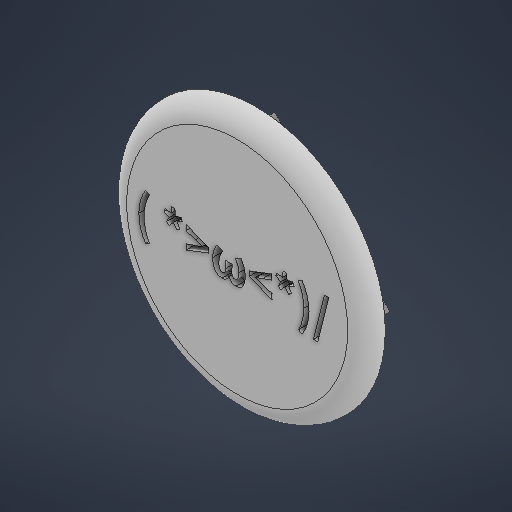
# Autodesk Inventor part: Part10
Saved by Autodesk Inventor 2026 (Build 300175000, 175)
## iProperties
Created: 2025-10-26
Part Number: Part10
Material: 一般
Document SubType Name: Modeling
Designer: masak
Density: 1 g/cm^3
Appearance: 既定
Author: masak
Autodesk Inventor part; units mm, degrees
ref_plane "YZ Plane" through (0, 0, 0) normal (1, 0, 0) x (0, 1, 0)
ref_plane "XZ Plane" through (0, 0, 0) normal (0, 1, 0) x (-1, 0, 0)
ref_plane "XY Plane" through (0, 0, 0) normal (0, 0, 1) x (1, 0, 0)
sketch "スケッチ1" plane through (0, 0, 0) normal (0, 0, 1) x (1, 0, 0)
  line L0 (23, 24.5) -> (3, 24.5) projected
  line L1 (23, 24.5) -> (3, 24.5) construction
  line L2 (23, 24.5) -> (3, 24.5)
  line L3 (23, 24.5) -> (3, 24.5)
  line L4 (23, 24.5) -> (3, 24.5)
  line L5 (23, 24.5) -> (3, 24.5) construction
  line L6 (13, 14.5) -> (3, 24.5) projected
  line L7 (3, 1.5) -> (13, 11.5) projected
  line L8 (11.5, 13) -> (1.5, 3) projected
  line L9 (1.5, 23) -> (11.5, 13) projected
  line L10 (1.5, 3) -> (1.5, 23) projected
  line L11 (0, 0) -> (0, 26) projected
  line L12 (0, 26) -> (50.5, 26) projected
  line L13 (50.5, 0) -> (0, 0) projected
  line L14 (0, 0) -> (-26, 0)
  line L15 (-26, 0) -> (-26, 26)
  line L16 (-26, 26) -> (0, 26)
  line L17 (0, 26) -> (0, 0)
  line L18 (-26, 0) -> (0, 26)
  line L19 (0, 0) -> (-26, 26)
  circle A0 centre (-13, 13) radius 27.5
  dimension "d0" = 26
  constraints: 18 end point, 2 parallel, 2 perpendicular, 1 centre point, 1 coincident, 1 horizontal, 1 midpoint
  measures "d0" distance of L15.end L16.end
extrude "押し出し1" add sketch "スケッチ1" along normal blind 4 contours L8 L10 L9 | L19 L18 L11 | L11 L12 A0 L13 | L13 A0 L12 L16 L15 L14 | L14 L18 L19 | L18 L19 L16 | L15 L19 L18
sketch "スケッチ2" plane through (-13, 13, 0) normal (0, 0, -1) x (-1, 0, 0)
  line L0 (-24.5, 0) -> (-14.5, 10) projected
  line L1 (-14.5, 10) -> (-14.5, -10) projected
  line L2 (-14.5, -10) -> (-24.5, 0) projected
  line L3 (-14.5, 10) -> (-14.5, -10)
  line L4 (-24.5, 0) -> (-14.5, 10)
  line L5 (-24.5, 0) -> (-14.5, -10)
  line L6 (-10, -14.5) -> (10, -14.5)
  line L7 (0, -24.5) -> (-10, -14.5)
  line L8 (0, -24.5) -> (10, -14.5)
  line L9 (14.5, -10) -> (14.5, 10)
  line L10 (24.5, 0) -> (14.5, -10)
  line L11 (24.5, 0) -> (14.5, 10)
  line L12 (10, 14.5) -> (-10, 14.5)
  line L13 (0, 24.5) -> (10, 14.5)
  line L14 (0, 24.5) -> (-10, 14.5)
  point P0 (-13, -13)
  point P1 (0, 0)
  dimension "d5" = 360
  constraints: 24 end point, 1 perpendicular, 1 vertical, 25 other
fillet "フィレット1" radius 4 1 edges at (-40.5, 13, 4)
extrude "押し出し2" add sketch "スケッチ2" along normal blind 4
sketch "スケッチ3" plane through (-13, 13, 4) normal (0, 0, 1) x (1, 0, 0)
  line L0 (-21.7114, 4.3311) -> (23.7979, 4.3311) construction
  line L1 (23.7979, 4.3311) -> (23.7979, -14.3854) construction
  line L2 (23.7979, -14.3854) -> (-21.7114, -14.3854) construction
  line L3 (-21.7114, -14.3854) -> (-21.7114, 4.3311) construction
  line L4 (-19.5093, -5.4449) -> (-18.6418, -5.0778)
  spline S0 degree 2 poles (-18.6418, -5.0778) (-19.229, -4.0369) (-19.7895, -1.728) (-19.7895, -0.5535) knots 0 0 0 1 2 2 2
  spline S1 degree 2 poles (-19.7895, -0.5535) (-19.7895, 0.6076) (-19.229, 2.9164) (-18.6418, 3.9574) knots 0 0 0 1 2 2 2
  line L5 (-18.6418, 3.9574) -> (-19.5093, 4.3244)
  spline S2 degree 2 poles (-19.5093, 4.3244) (-20.1766, 3.2434) (-20.9039, 0.8478) (-20.9106, -0.5535) knots 0 0 0 1 2 2 2
  spline S3 degree 2 poles (-20.9106, -0.5535) (-20.9039, -1.9682) (-20.1766, -4.3572) (-19.5093, -5.4449) knots 0 0 0 1 2 2 2
  line L6 (-14.4444, 0.4074) -> (-13.617, 1.3549)
  line L7 (-13.617, 1.3549) -> (-12.7895, 0.4074)
  line L8 (-12.7895, 0.4074) -> (-12.1823, 0.8411)
  line L9 (-12.1823, 0.8411) -> (-12.8229, 1.9155)
  line L10 (-12.8229, 1.9155) -> (-11.6952, 2.416)
  line L11 (-11.6952, 2.416) -> (-11.922, 3.1166)
  line L12 (-11.922, 3.1166) -> (-13.1299, 2.843)
  line L13 (-13.1299, 2.843) -> (-13.2433, 4.0909)
  line L14 (-13.2433, 4.0909) -> (-13.984, 4.0909)
  line L15 (-13.984, 4.0909) -> (-14.1041, 2.8564)
  line L16 (-14.1041, 2.8564) -> (-15.3119, 3.1166)
  line L17 (-15.3119, 3.1166) -> (-15.5388, 2.416)
  line L18 (-15.5388, 2.416) -> (-14.4177, 1.9155)
  line L19 (-14.4177, 1.9155) -> (-15.0383, 0.8411)
  line L20 (-15.0383, 0.8411) -> (-14.4444, 0.4074)
  line L21 (-10.8744, -2.3486) -> (-6.0364, -0.4801)
  line L22 (-6.0364, -0.4801) -> (-6.0364, 0.5141)
  line L23 (-6.0364, 0.5141) -> (-10.881, 2.3826)
  line L24 (-10.881, 2.3826) -> (-10.881, 1.2282)
  line L25 (-10.881, 1.2282) -> (-8.8858, 0.5475)
  line L26 (-8.8858, 0.5475) -> (-7.4444, 0.0404)
  line L27 (-7.4444, 0.0404) -> (-7.4444, 0.0003)
  line L28 (-7.4444, 0.0003) -> (-8.8858, -0.5135)
  line L29 (-8.8858, -0.5135) -> (-10.881, -1.1941)
  line L30 (-10.881, -1.1941) -> (-10.8744, -2.3486)
  spline S4 degree 2 poles (-3.2137, -3.6698) (-2.74, -3.6765) (-1.9926, -3.2094) (-1.779, -2.6756) knots 0 0 0 1 2 2 2
  line L31 (-1.779, -2.6756) -> (-1.739, -2.6756)
  spline S5 degree 2 poles (-1.739, -2.6756) (-1.5188, -3.2094) (-0.7047, -3.6765) (-0.2309, -3.6698) knots 0 0 0 1 2 2 2
  spline S6 degree 2 poles (-0.2309, -3.6698) (0.6966, -3.6632) (1.7043, -2.2218) (1.7109, -0.8672) knots 0 0 0 1 2 2 2
  spline S7 degree 2 poles (1.7109, -0.8672) (1.7043, -0.0264) (1.2505, 1.2949) (0.8701, 1.8821) knots 0 0 0 1 2 2 2
  line L32 (0.8701, 1.8821) -> (-0.3911, 1.4017)
  spline S8 degree 2 poles (-0.3911, 1.4017) (-0.1241, 0.9813) (0.1895, 0.2539) (0.323, -0.5002) (0.323, -0.9472) knots 0 0 0 1 2 3 3 3
  spline S9 degree 2 poles (0.323, -0.9472) (0.3163, -1.7347) (-0.0908, -2.5354) (-0.4311, -2.5354) knots 0 0 0 1 2 2 2
  spline S10 degree 2 poles (-0.4311, -2.5354) (-0.7647, -2.5421) (-1.1451, -2.0616) (-1.1451, -1.4677) knots 0 0 0 1 2 2 2
  spline S11 degree 2 poles (-1.1451, -1.4677) (-1.1451, -1.1207) (-1.0784, -0.4935) (-1.025, -0.0531) knots 0 0 0 1 2 2 2
  line L33 (-1.025, -0.0531) -> (-2.4931, -0.0531)
  spline S12 degree 2 poles (-2.4931, -0.0531) (-2.433, -0.4935) (-2.3796, -1.1207) (-2.3796, -1.4677) knots 0 0 0 1 2 2 2
  spline S13 degree 2 poles (-2.3796, -1.4677) (-2.3863, -2.0283) (-2.7933, -2.5421) (-3.147, -2.5354) knots 0 0 0 1 2 2 2
  spline S14 degree 2 poles (-3.147, -2.5354) (-3.5074, -2.5288) (-3.9011, -1.8014) (-3.9011, -1.1675) knots 0 0 0 1 2 2 2
  spline S15 degree 2 poles (-3.9011, -1.1675) (-3.9011, -0.4735) (-3.4673, 0.7344) (-3.0603, 1.375) knots 0 0 0 1 2 2 2
  line L34 (-3.0603, 1.375) -> (-4.3548, 1.8821)
  spline S16 degree 2 poles (-4.3548, 1.8821) (-4.7285, 1.2815) (-5.209, -0.1799) (-5.2157, -0.9005) knots 0 0 0 1 2 2 2
  spline S17 degree 2 poles (-5.2157, -0.9005) (-5.2023, -2.2618) (-4.128, -3.6632) (-3.2137, -3.6698) knots 0 0 0 1 2 2 2
  line L35 (7.3897, -2.3486) -> (7.3897, -1.1941)
  line L36 (7.3897, -1.1941) -> (5.4078, -0.5135)
  line L37 (5.4078, -0.5135) -> (3.9598, 0.0003)
  line L38 (3.9598, 0.0003) -> (3.9598, 0.0404)
  line L39 (3.9598, 0.0404) -> (5.4011, 0.5475)
  line L40 (5.4011, 0.5475) -> (7.383, 1.2282)
  line L41 (7.383, 1.2282) -> (7.383, 2.3826)
  line L42 (7.383, 2.3826) -> (2.5451, 0.5141)
  line L43 (2.5451, 0.5141) -> (2.5451, -0.4801)
  line L44 (2.5451, -0.4801) -> (7.3897, -2.3486)
  line L45 (9.3048, 0.4074) -> (10.1323, 1.3549)
  line L46 (10.1323, 1.3549) -> (10.9598, 0.4074)
  line L47 (10.9598, 0.4074) -> (11.567, 0.8411)
  line L48 (11.567, 0.8411) -> (10.9264, 1.9155)
  line L49 (10.9264, 1.9155) -> (12.0541, 2.416)
  line L50 (12.0541, 2.416) -> (11.8272, 3.1166)
  line L51 (11.8272, 3.1166) -> (10.6194, 2.843)
  line L52 (10.6194, 2.843) -> (10.506, 4.0909)
  line L53 (10.506, 4.0909) -> (9.7653, 4.0909)
  line L54 (9.7653, 4.0909) -> (9.6452, 2.8564)
  line L55 (9.6452, 2.8564) -> (8.4374, 3.1166)
  line L56 (8.4374, 3.1166) -> (8.2105, 2.416)
  line L57 (8.2105, 2.416) -> (9.3315, 1.9155)
  line L58 (9.3315, 1.9155) -> (8.7109, 0.8411)
  line L59 (8.7109, 0.8411) -> (9.3048, 0.4074)
  spline S18 degree 2 poles (13.8625, -5.4449) (14.5365, -4.3572) (15.2705, -1.9682) (15.2772, -0.5535) knots 0 0 0 1 2 2 2
  spline S19 degree 2 poles (15.2772, -0.5535) (15.2705, 0.8478) (14.5365, 3.2434) (13.8625, 4.3244) knots 0 0 0 1 2 2 2
  line L60 (13.8625, 4.3244) -> (13.0084, 3.9574)
  spline S20 degree 2 poles (13.0084, 3.9574) (13.5956, 2.9164) (14.1561, 0.6076) (14.1561, -0.5535) knots 0 0 0 1 2 2 2
  spline S21 degree 2 poles (14.1561, -0.5535) (14.1561, -1.728) (13.5956, -4.0369) (13.0084, -5.0778) knots 0 0 0 1 2 2 2
  line L61 (13.0084, -5.0778) -> (13.8625, -5.4449)
  line L62 (16.2114, -5.2513) -> (17.139, -5.2513)
  line L63 (17.139, -5.2513) -> (19.4745, 4.0709)
  line L64 (19.4745, 4.0709) -> (18.5603, 4.0709)
  line L65 (18.5603, 4.0709) -> (16.2114, -5.2513)
  point P0 (13, -13)
  constraints: 2 other
extrude "押し出し3" cut sketch "スケッチ3" against normal blind 2
